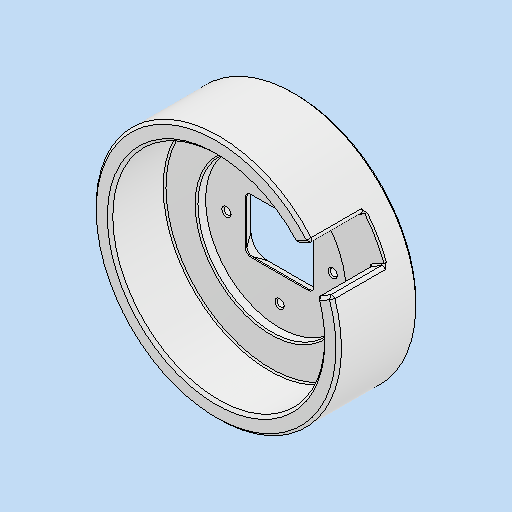
# Autodesk Inventor part: QHY183-flange-adapter
Saved by Autodesk Inventor 2025 (Build 290162000, 162)
## iProperties
Created: 2025-02-17
Part Number: QHY183-flange-adapter
Material: ABS Plastic
Document SubType Name: Modeling
Designer: kuzmin
Density: 1.06 g/cm^3
Appearance: Smooth - White
Author: kuzmin
Autodesk Inventor part; units mm, degrees
ref_plane "YZ Plane" through (0, 0, 0) normal (1, 0, 0) x (0, 1, 0)
ref_plane "XZ Plane" through (0, 0, 0) normal (0, 1, 0) x (-1, 0, 0)
ref_plane "XY Plane" through (0, 0, 0) normal (0, 0, 1) x (1, 0, 0)
sketch "Sketch1" plane through (0, 0, 0) normal (0, 1, 0) x (-1, 0, 0)
  line L0 (0, 0) -> (0, 33.2322)
  line L1 (10, 0) -> (45, 0)
  line L2 (45, 0) -> (45, 5.3)
  line L3 (27.15, 9.3) -> (27.15, 6)
  line L4 (27.15, 6) -> (10, 6)
  line L5 (10, 6) -> (10, 0)
  line L6 (27.15, 9.3) -> (38.9, 9.3)
  line L7 (38.9, 9.3) -> (38.9, 29.3)
  line L8 (38.9, 29.3) -> (45, 29.3)
  line L9 (45, 29.3) -> (45, 5.3)
  point P0 (0, 16.6161)
  dimension "d0" = 54.3
  dimension "d1" = 20
  dimension "d2" = 3.3
  dimension "d3" = 6
  dimension "d4" = 90
  dimension "d6" = 77.8
  dimension "d7" = 20
  constraints: 20 end point, 6 perpendicular, 2 horizontal, 1 horizontal alignment, 1 midpoint, 1 vertical
  measures "d0" diameter of L3 point (0, 16.616)
  measures "d1" diameter of L5 L0
  measures "d2" distance of L3.start L3.end
  measures "d3" distance of L4.end L1.start
  measures "d4" diameter of L2 L0
  measures "d6" diameter of L7 L0
  measures "d7" distance of L6.end L7.end
revolve "Revolution1" add sketch "Sketch1" angle 360 about axis through (0, 0, 0) along (0, 0, 1)
sketch "Sketch2" plane through (0, 0, 0) normal (0, 0, -1) x (-1, 0, 0)
  line L0 (-12.5, 10) -> (12.5, 10)
  line L1 (12.5, 10) -> (12.5, -10)
  line L2 (12.5, -10) -> (-12.5, -10)
  line L3 (-12.5, -10) -> (-12.5, 10)
  point P0 (0, 0)
  point P1 (12.5, 0)
  point P2 (0, 10)
  dimension "d8" = 20
  dimension "d9" = 25
  constraints: 8 end point, 2 midpoint, 2 parallel, 1 horizontal, 1 horizontal alignment, 1 perpendicular, 1 vertical alignment
  measures "d8" distance of L0.end L1.end
  measures "d9" distance of L0.start L0.end
extrude "Extrusion1" cut sketch "Sketch2" against normal through all
fillet "Fillet1" radius 2 4 edges at (-12.5, -10, 3) (12.5, -10, 3) (12.5, 10, 3) (-12.5, 10, 3)
sketch "Sketch3" plane through (0, 0, 0) normal (0, 0, 1) x (1, 0, 0)
  circle A0 centre (0, 0) radius 19.5 construction
  point P0 (0, -19.5)
  point P1 (-19.5, 0)
  point P2 (0, 19.5)
  point P3 (19.5, 0)
  dimension "d68" = 39
  constraints: 3 vertical alignment, 2 horizontal alignment, 1 coincident, 2 other
hole "CameraMounts" at (0, -19.5, 0) at (-19.5, 0, 0) at (0, 19.5, 0) at (19.5, 0, 0) direction (0, 0, 1) diameter 2.6 end through all counterbore diameter 4.5 counterbore depth 3
sketch "Sketch8" plane through (-19.5, 0, 3) normal (0, 0, -1) x (-1, 0, 0)
  circle A0 centre (0, 0) radius 2.25 projected
  circle A1 centre (0, 0) radius 1.3 projected
  line L0 (1.8364, 1.3) -> (-1.8364, 1.3)
  line L1 (1.8364, -1.3) -> (-1.8364, -1.3)
  line L2 (-1.3, -1.8364) -> (-1.3, 1.8364)
  line L3 (1.3, 1.8364) -> (1.3, -1.8364)
  point P0 (-19.5, 0)
  constraints: 8 end point, 4 tangent, 1 horizontal, 1 parallel, 1 perpendicular, 1 vertical, 9 other
extrude "Extrusion4" add sketch "Sketch8" along normal blind 0.28 contours L0 L3 A0 | A0 L3 L1 | L3 L0 L2 A0 | A0 L2 L1 L3 | L2 L0 A0 | A0 L1 L2
extrude "Extrusion5" add sketch "Sketch8" along normal blind 0.56 contours A0 L1 L3 L0 | L0 L3 A0 | A0 L3 L1 | L2 L0 A0 | A0 L1 L2 | L0 L2 L1 A0
pattern_circular "Circular Pattern1" count 4 over 360 about axis through (0, 0, -10) along (0, 0, 1) of "Extrusion5", "Extrusion4"
sketch "Sketch4" plane through (0, 0, 9.3) normal (0, 0, 1) x (1, 0, 0)
  line L0 (0, 0) -> (38.5537, 22.259) construction
  line L1 (29.7308, 8.5048) -> (22.2308, 21.4952)
  line L2 (22.2308, 21.4952) -> (35.2211, 28.9952)
  line L3 (35.2211, 28.9952) -> (42.7211, 16.0048)
  line L4 (42.7211, 16.0048) -> (29.7308, 8.5048)
  line L5 (0, 0) -> (19.5, 0) construction
  point P0 (25.9808, 15)
  dimension "d24" = 30
  dimension "d25" = 45
  dimension "d26" = 15
  dimension "d69" = 30
  constraints: 12 end point, 4 perpendicular, 1 horizontal, 1 midpoint, 1 point on line
  measures "d24" distance from line of L0.start L1
  measures "d25" distance from line of L0.start L3
  measures "d26" distance of L2.end L3.end
  measures "d69" angle of L5 L0
extrude "BoltCutOut" cut sketch "Sketch4" along normal through all
fillet "Fillet2" radius 1 4 edges at (29.3063, 25.5803, 19.3) (34.6761, 28.6805, 19.3) (36.8063, 12.5899, 19.3) (42.1761, 15.6901, 19.3)
chamfer "Chamfer2" distance 1 angle 45 9 edges at (-33.6884, -19.45, 29.3) (37.0786, 12.4916, 29.3) (39.3243, 14.0436, 29.3) (41.9887, 15.1606, 29.3) (-15.8103, 42.1312, 29.3) (7.3735, -44.3918, 29.3) (34.1238, 28.7829, 29.3) (31.8243, 27.034, 29.3) (29.3574, 25.8652, 29.3)
chamfer "Chamfer3" distance 0.5 angle 45 8 edges at (-33.6884, -19.45, 9.3) (37.0786, 12.4916, 9.3) (39.3243, 14.0436, 9.3) (41.9887, 15.1606, 9.3) (29.3574, 25.8652, 9.3) (31.8243, 27.034, 9.3) (34.1238, 28.7829, 9.3) (27.15, 0, 9.3)
chamfer "Chamfer4" distance 1 angle 45 1 edges at (45, 0, 0)
chamfer "Window" distance 4 angle 54 8 edges at (0, 10, 0) (-11.9142, 9.4142, 0) (-12.5, 0, 0) (-11.9142, -9.4142, 0) (0, -10, 0) (11.9142, -9.4142, 0) (12.5, 0, 0) (11.9142, 9.4142, 0) measured on face at (13, 0, 0) measured on face at (0, 10.5, 0) measured on face at (-12.2678, -9.7678, 0) measured on face at (0, -10.5, 0) measured on face at (12.2678, 9.7678, 0) measured on face at (-12.2678, 9.7678, 0) measured on face at (-13, 0, 0) measured on face at (12.2678, -9.7678, 0)
sketch "Sketch7" plane through (0, 0, 0) normal (0, 0, -1) x (-1, 0, 0)
  circle A0 centre (0, 0) radius 37.5 construction
  point P0 (0, 37.5)
  point P1 (0, -37.5)
  point P2 (37.5, 0)
  point P3 (-37.5, 0)
  dimension "d54" = 75
  constraints: 4 point on circle, 2 horizontal alignment, 2 vertical alignment, 1 centre point, 1 coincident
  measures "d54" diameter of A0
hole "PlateMounts" at (0, 37.5, 0) at (0, -37.5, 0) at (-37.5, 0, 0) at (37.5, 0, 0) direction (0, 0, 1) diameter 4.6 depth 6 tip angle 80 counterbore diameter 5.1 counterbore depth 1
chamfer "Chamfer6" distance 0.5 angle 45 1 edges at (38.9711, 22.5, 9.3)
chamfer "Chamfer8" distance 0.4 angle 45 8 edges at (0, 17.25, 0) (-19.5, -2.25, 0) (0, -21.75, 0) (19.5, -2.25, 0) (0, 18.2, 6) (19.5, -1.3, 6) (0, -20.8, 6) (-19.5, -1.3, 6)
sketch "Sketch9" plane through (0, 0, 0) normal (0, 0, -1) x (-1, 0, 0)
  circle A0 centre (0, 0) radius 30
  circle A1 centre (0, 0) radius 32
  dimension "d80" = 60
  dimension "d81" = 64
  constraints: 2 centre point, 2 coincident
  measures "d80" diameter of A0
  measures "d81" diameter of A1
extrude "LightSeam" cut sketch "Sketch9" against normal blind 3
chamfer "Chamfer9" distance 0.4 angle 45 4 edges at (30, 0, 0) (32, 0, 0) (32, 0, 3) (30, 0, 3)
